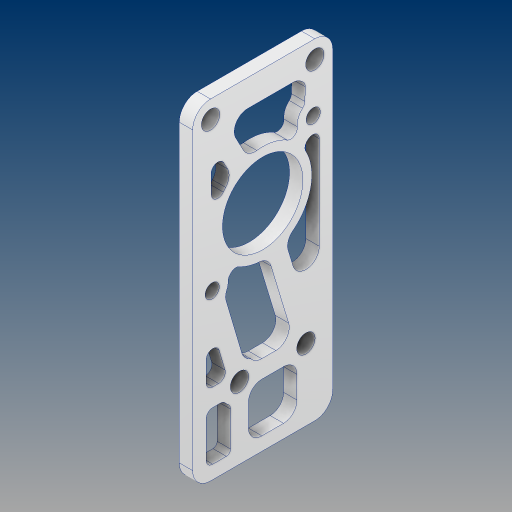
# Autodesk Inventor part: INTK_008_EncoderBracket
Saved by Autodesk Inventor 2024.3 (Build 283343000, 343)
## iProperties
Created: 2024-08-04
Part Number: INTK_008_EncoderBracket
Material: Aluminum 6061
Document SubType Name: Modeling
Designer: Kenji
Density: 2.7 g/cm^3
Appearance: Aluminum - Flat
Author: Kenji
Autodesk Inventor part; units mm, degrees
ref_plane "YZ Plane" through (0, 0, 0) normal (1, 0, 0) x (0, 1, 0)
ref_plane "XZ Plane" through (0, 0, 0) normal (0, 1, 0) x (-1, 0, 0)
ref_plane "XY Plane" through (0, 0, 0) normal (0, 0, 1) x (1, 0, 0)
sketch "Sketch1" plane through (0, 0, 0) normal (1, 0, 0) x (0, 1, 0)
  line L0 (0, 0) -> (457.2, 0) construction
  line L1 (457.2, 0) -> (457.2, 25.4) construction
  line L2 (457.2, 25.4) -> (0, 25.4) construction
  line L3 (0, 25.4) -> (0, 0) construction
  line L4 (0, 0) -> (25.4, 0) construction
  line L5 (25.4, 0) -> (25.4, -279.4) construction
  line L6 (25.4, -279.4) -> (0, -279.4) construction
  line L7 (0, -279.4) -> (0, 0) construction
  line L8 (0, 0) -> (25.4, 0) construction
  line L9 (25.4, 0) -> (25.4, -19.05) construction
  line L10 (25.4, -19.05) -> (0, -19.05) construction
  line L11 (0, -19.05) -> (0, 0) construction
  line L12 (25.4, -279.4) -> (0, -279.4) construction
  line L13 (0, -279.4) -> (0, -260.35) construction
  line L14 (0, -260.35) -> (25.4, -260.35) construction
  line L15 (25.4, -260.35) -> (25.4, -279.4) construction
  circle A0 centre (101.6254, -38.1) radius 14.2875
  line L16 (83.6649, -20.1395) -> (119.5859, -56.0605) construction
  line L17 (101.6254, -38.1) -> (101.6254, -52.3875) construction
  circle A1 centre (119.5859, -56.0605) radius 2.5019
  circle A2 centre (83.6649, -20.1395) radius 2.5019
  line L18 (25.4, -20.32) -> (57.15, -20.32) construction
  line L19 (57.15, -20.32) -> (57.15, -39.37) construction
  line L20 (57.15, -39.37) -> (25.4, -39.37) construction
  line L21 (25.4, -39.37) -> (25.4, -20.32) construction
  circle A3 centre (50.8, -29.845) radius 3.2512
  circle A4 centre (136.6774, -19.558) radius 6.35 construction
  circle A5 centre (136.6774, -19.558) radius 3.2512
  line L22 (72.9234, -13.208) -> (130.3274, -13.208) construction
  line L23 (130.3274, -13.208) -> (130.3274, -62.992) construction
  line L24 (130.3274, -62.992) -> (72.9234, -62.992) construction
  line L25 (72.9234, -62.992) -> (72.9234, -13.208) construction
  line L26 (25.4, -43.942) -> (57.15, -43.942) construction
  line L27 (57.15, -43.942) -> (57.15, -62.992) construction
  line L28 (57.15, -62.992) -> (25.4, -62.992) construction
  line L29 (25.4, -62.992) -> (25.4, -43.942) construction
  circle A6 centre (50.8, -53.467) radius 3.2512
  circle A7 centre (136.6774, -56.642) radius 6.35 construction
  circle A8 centre (136.6774, -56.642) radius 3.2512
  line L30 (136.6774, -62.992) -> (31.75, -62.992)
  line L31 (25.4, -56.642) -> (25.4, -19.558)
  line L32 (31.75, -13.208) -> (136.6774, -13.208)
  arc A9 (31.75, -13.208) -> (25.4, -19.558) centre (31.75, -19.558) ccw
  arc A10 (25.4, -56.642) -> (31.75, -62.992) centre (31.75, -56.642) ccw
  line L33 (143.0274, -19.558) -> (143.0274, -56.642)
  arc A11 (136.6774, -62.992) -> (143.0274, -56.642) centre (136.6774, -56.642) ccw
  arc A12 (143.0274, -19.558) -> (136.6774, -13.208) centre (136.6774, -19.558) ccw
  point P0 (83.6649, -17.6376)
  point P1 (101.6254, -38.1)
  point P2 (101.6254, -62.992)
  point P3 (25.4, -62.992)
  point P4 (25.4, -13.208)
  dimension "d7" = 28.575
  dimension "d14" = 5.0038
  dimension "d0" = 457.2
  dimension "d1" = 25.4
  dimension "d2" = 25.4
  dimension "d3" = 279.4
  dimension "d5" = 19.05
  dimension "d8" = 101.6254
  dimension "d9" = 38.1
  dimension "d10" = 50.8
  dimension "d11" = 25.4
  dimension "d12" = 45
  dimension "d13" = 5.0038
  dimension "d15" = 31.75
  dimension "d16" = 19.05
  dimension "d18" = 6.5024
  dimension "d19" = 9.525
  dimension "d20" = 6.35
  dimension "d27" = 12.7
  dimension "d28" = 6.5024
  dimension "d34" = 49.784
  dimension "d35" = 57.404
  dimension "d36" = 24.892
  dimension "d37" = 28.702
  dimension "d46" = 31.75
  dimension "d47" = 19.05
  dimension "d48" = 6.5024
  dimension "d49" = 9.525
  dimension "d50" = 6.35
  dimension "d51" = 12.7
  dimension "d52" = 6.5024
  dimension "d53" = 6.35
  dimension "d128" = 29.845
  dimension "d129" = 19.05
  dimension "d130" = 53.467
  constraints: 68 end point, 14 parallel, 12 point on circle, 12 point on line, 11 centre point, 10 tangent, 8 perpendicular, 7 horizontal, 6 coincident, 3 equal radius, 3 vertical alignment, 2 collinear, 2 midpoint, 2 vertical, 4 other
  measures "d0" distance of L2.end L1.end
  measures "d1" distance of L1.end L0.end
  measures "d2" distance of L5.end L6.end
  measures "d3" distance of L4.end L5.end
  measures "d5" distance of L12.end L13.end
  measures "d8" distance from line of L7 point (101.625, -38.1)
  measures "d9" distance from line of L0 point (101.625, -38.1)
  measures "d10" distance of L16.start L16.end
  measures "d11" distance of L16.end L17.start
  measures "d12" angle of L17 L16
  measures "d13" diameter of A1
  measures "d15" distance of L19.end L20.end
  measures "d16" distance of L18.end L19.end
  measures "d18" diameter of A3
  measures "d19" distance from line of L18 A3.centre
  measures "d20" distance from line of L19 A3.centre
  measures "d27" diameter of A4
  measures "d28" diameter of A5
  measures "d34" distance of L22.end L23.end
  measures "d35" distance between parallel lines of L25 L23
  measures "d36" distance of point (101.625, -62.992) point (101.625, -38.1)
  measures "d37" distance from line of L25 point (101.625, -38.1)
  measures "d46" distance of L27.end L28.end
  measures "d47" distance of L26.end L27.end
  measures "d48" diameter of A6
  measures "d49" distance from line of L26 A6.centre
  measures "d50" distance from line of L27 A6.centre
  measures "d51" diameter of A7
  measures "d52" diameter of A8
  measures "d53" radius of A9
  measures "d128" distance from line of L0 A3.centre
  measures "d129" distance between parallel lines of L0 L10
  measures "d130" distance from line of L0 A6.centre
extrude "Extrusion2" add sketch "Sketch1" along normal blind 4.7625
sketch "Sketch2" plane through (4.7625, 0, 0) normal (1, 0, 0) x (0, 0, -1)
  line L0 (13.208, 136.6774) -> (13.208, 31.75) construction
  arc A0 (13.208, 31.75) -> (19.558, 25.4) centre (19.558, 31.75) ccw construction
  line L1 (19.558, 25.4) -> (56.642, 25.4) construction
  arc A1 (56.642, 25.4) -> (62.992, 31.75) centre (56.642, 31.75) ccw construction
  line L2 (62.992, 31.75) -> (62.992, 136.6774) construction
  arc A2 (62.992, 136.6774) -> (56.642, 143.0274) centre (56.642, 136.6774) ccw construction
  line L3 (56.642, 143.0274) -> (19.558, 143.0274) construction
  arc A3 (19.558, 143.0274) -> (13.208, 136.6774) centre (19.558, 136.6774) ccw construction
  circle A4 centre (38.1, 101.6254) radius 14.2875 construction
  circle A5 centre (56.0605, 119.5859) radius 2.5019 construction
  circle A6 centre (20.1395, 83.6649) radius 2.5019 construction
  circle A7 centre (29.845, 50.8) radius 3.2512 construction
  circle A8 centre (53.467, 50.8) radius 3.2512 construction
  circle A9 centre (56.642, 136.6774) radius 3.2512 construction
  circle A10 centre (19.558, 136.6774) radius 3.2512 construction
  line L4 (19.558, 138.2522) -> (56.642, 138.2522) construction
  arc A11 (58.2168, 136.6774) -> (56.642, 138.2522) centre (56.642, 136.6774) ccw construction
  line L5 (58.2168, 136.6774) -> (58.2168, 31.75) construction
  arc A12 (56.642, 30.1752) -> (58.2168, 31.75) centre (56.642, 31.75) ccw construction
  line L6 (56.642, 30.1752) -> (19.558, 30.1752) construction
  arc A13 (17.9832, 31.75) -> (19.558, 30.1752) centre (19.558, 31.75) ccw construction
  line L7 (17.9832, 31.75) -> (17.9832, 136.6774) construction
  arc A14 (19.558, 138.2522) -> (17.9832, 136.6774) centre (19.558, 136.6774) ccw construction
  circle A15 centre (19.558, 136.6774) radius 6.4262 construction
  circle A16 centre (56.642, 136.6774) radius 6.4262 construction
  circle A17 centre (56.0605, 119.5859) radius 5.6769 construction
  circle A18 centre (38.1, 101.6254) radius 17.4625 construction
  circle A19 centre (20.1395, 83.6649) radius 5.6769 construction
  circle A20 centre (29.845, 50.8) radius 6.4262 construction
  circle A21 centre (53.467, 50.8) radius 6.4262 construction
  line L8 (22.5628, 130.997) -> (29.9347, 117.0613) construction
  line L9 (56.4235, 130.2549) -> (56.2535, 125.2595) construction
  line L10 (52.0463, 115.5717) -> (50.4479, 113.9733) construction
  line L11 (53.2364, 129.9526) -> (53.0859, 125.5295)
  line L12 (19.6285, 130.2516) -> (20.0772, 89.3414) construction
  line L13 (28.5365, 126.4943) -> (31.1955, 121.4677)
  line L14 (25.9842, 136.6774) -> (50.2158, 136.6774) construction
  line L15 (32.7576, 133.5024) -> (48.7511, 133.5024)
  arc A22 (46.8385, 116.7442) -> (35.9928, 118.9603) centre (38.1, 101.6254) ccw
  arc A23 (52.2868, 123.827) -> (50.4099, 119.0407) centre (56.0605, 119.5859) ccw
  arc A24 (24.977, 133.2233) -> (25.1451, 133.5024) centre (19.558, 136.6774) ccw
  arc A25 (52.115, 132.1164) -> (52.4191, 131.8335) centre (56.642, 136.6774) ccw
  arc A26 (52.115, 132.1164) -> (48.7511, 133.5024) centre (48.7511, 128.7272) ccw
  arc A27 (32.7576, 133.5024) -> (28.5365, 126.4943) centre (32.7576, 128.7272) ccw
  arc A28 (31.1955, 121.4677) -> (35.9928, 118.9603) centre (35.4166, 123.7006) ccw
  circle A29 centre (48.0333, 118.8113) radius 2.3876 construction
  arc A30 (46.8385, 116.7442) -> (50.4099, 119.0407) centre (48.0333, 118.8113) ccw
  circle A31 centre (50.8502, 130.0338) radius 2.3876 construction
  circle A32 centre (50.6997, 125.6107) radius 2.3876 construction
  arc A33 (53.2364, 129.9526) -> (52.4191, 131.8335) centre (50.8502, 130.0338) ccw
  arc A34 (52.2868, 123.827) -> (53.0859, 125.5295) centre (50.6997, 125.6107) ccw
  line L16 (21.7473, 78.2204) -> (28.0249, 56.9631) construction
  line L17 (47.0408, 50.8) -> (36.2712, 50.8) construction
  line L18 (51.6072, 56.9512) -> (43.1538, 84.9102) construction
  line L19 (23.4188, 50.8) -> (17.9832, 50.8) construction
  line L20 (29.845, 44.3738) -> (29.845, 30.1752) construction
  line L21 (53.467, 44.3738) -> (53.467, 30.1752) construction
  line L22 (45.5168, 47.625) -> (37.7952, 47.625)
  line L23 (33.02, 42.8498) -> (33.02, 34.9504)
  line L24 (50.292, 42.8498) -> (50.292, 34.9504)
  line L25 (20.6386, 101.4339) -> (19.9447, 101.4263) construction
  line L26 (24.2401, 121.0363) -> (25.5825, 118.4985)
  arc A35 (24.9558, 113.1219) -> (24.1124, 112.0794) centre (38.1, 101.6254) ccw
  line L27 (19.7421, 119.8937) -> (19.8124, 113.4825)
  circle A36 centre (22.1296, 119.9199) radius 2.3876 construction
  arc A37 (24.9558, 113.1219) -> (25.5825, 118.4985) centre (21.3615, 116.2657) ccw
  arc A38 (24.2401, 121.0363) -> (19.7421, 119.8937) centre (22.1296, 119.9199) ccw
  circle A39 centre (22.1999, 113.5087) radius 2.3876 construction
  arc A40 (19.8124, 113.4825) -> (24.1124, 112.0794) centre (22.1999, 113.5087) ccw
  arc A41 (33.02, 45.2129) -> (35.4321, 47.625) centre (29.845, 50.8) ccw construction
  line L28 (37.7952, 30.1752) -> (45.5168, 30.1752)
  arc A42 (33.02, 45.2129) -> (35.4321, 47.625) centre (29.845, 50.8) ccw construction
  arc A43 (47.8799, 47.625) -> (50.292, 45.2129) centre (53.467, 50.8) ccw construction
  arc A44 (37.7952, 47.625) -> (33.02, 42.8498) centre (37.7952, 42.8498) ccw
  arc A45 (50.292, 42.8498) -> (45.5168, 47.625) centre (45.5168, 42.8498) ccw
  arc A46 (33.02, 34.9504) -> (37.7952, 30.1752) centre (37.7952, 34.9504) ccw
  arc A47 (45.5168, 30.1752) -> (50.292, 34.9504) centre (45.5168, 34.9504) ccw
  line L29 (23.0204, 47.625) -> (20.3454, 47.625)
  line L30 (26.67, 43.9754) -> (26.67, 31.6738)
  line L31 (17.9832, 45.2628) -> (17.9832, 32.5374)
  line L32 (20.3454, 30.1752) -> (25.1714, 30.1752)
  circle A48 centre (25.1714, 31.6738) radius 1.4986 construction
  arc A49 (25.1714, 30.1752) -> (26.67, 31.6738) centre (25.1714, 31.6738) ccw
  arc A50 (17.9832, 32.5374) -> (20.3454, 30.1752) centre (20.3454, 32.5374) ccw
  arc A51 (24.8547, 46.7511) -> (25.7961, 45.8097) centre (29.845, 50.8) ccw
  arc A52 (24.8547, 46.7511) -> (23.0204, 47.625) centre (23.0204, 45.2628) ccw
  arc A53 (26.67, 43.9754) -> (25.7961, 45.8097) centre (24.3078, 43.9754) ccw
  arc A54 (20.3454, 47.625) -> (17.9832, 45.2628) centre (20.3454, 45.2628) ccw
  line L33 (24.1537, 87.6791) -> (25.7521, 89.2775) construction
  line L34 (26.5133, 85.5486) -> (26.8713, 85.9066)
  line L35 (47.3285, 60.1322) -> (41.0713, 80.8273)
  line L36 (25.1062, 78.0566) -> (30.6551, 59.267)
  line L37 (42.7576, 53.975) -> (37.7359, 53.975)
  arc A55 (29.7071, 86.312) -> (36.844, 84.2081) centre (38.1, 101.6254) ccw
  arc A56 (25.3245, 81.3534) -> (25.8147, 83.8025) centre (20.1395, 83.6649) ccw
  arc A57 (34.372, 55.361) -> (32.9371, 56.4334) centre (29.845, 50.8) ccw
  arc A58 (48.8109, 55.2291) -> (47.8799, 53.975) centre (53.467, 50.8) ccw construction
  arc A59 (41.0713, 80.8273) -> (36.844, 84.2081) centre (36.5005, 79.4453) ccw
  arc A60 (42.7576, 53.975) -> (47.3285, 60.1322) centre (42.7576, 58.7502) ccw
  arc A61 (34.372, 55.361) -> (37.7359, 53.975) centre (37.7359, 58.7502) ccw
  arc A62 (30.6551, 59.267) -> (32.9371, 56.4334) centre (35.2348, 60.6194) ccw
  circle A63 centre (28.5596, 84.2183) radius 2.3876 construction
  arc A64 (25.3245, 81.3534) -> (25.1062, 78.0566) centre (29.6859, 79.4091) ccw
  circle A65 centre (28.2016, 83.8603) radius 2.3876 construction
  arc A66 (29.7071, 86.312) -> (26.8713, 85.9066) centre (28.5596, 84.2183) ccw
  arc A67 (26.5133, 85.5486) -> (25.8147, 83.8025) centre (28.2016, 83.8603) ccw
  line L38 (54.1409, 113.1762) -> (53.8188, 112.8541)
  line L39 (48.8708, 76.9724) -> (47.1496, 82.665)
  line L40 (58.2168, 111.4879) -> (58.2168, 78.3544)
  arc A68 (58.2168, 55.1284) -> (54.8892, 57.0669) centre (53.467, 50.8) ccw construction
  arc A69 (48.7957, 87.8217) -> (53.4134, 110.0183) centre (38.1, 101.6254) ccw
  arc A70 (48.7957, 87.8217) -> (47.1496, 82.665) centre (51.7204, 84.047) ccw
  arc A71 (48.8708, 76.9724) -> (58.2168, 78.3544) centre (53.4416, 78.3544) ccw
  circle A72 centre (55.5071, 111.1658) radius 2.3876 construction
  circle A73 centre (55.8292, 111.4879) radius 2.3876 construction
  arc A74 (58.2168, 111.4879) -> (54.1409, 113.1762) centre (55.8292, 111.4879) ccw
  arc A75 (53.8188, 112.8541) -> (53.4134, 110.0183) centre (55.5071, 111.1658) ccw
  line L41 (22.6109, 64.086) -> (24.7016, 57.0062)
  line L42 (22.4362, 53.975) -> (20.3454, 53.975)
  line L43 (17.9832, 63.417) -> (17.9832, 56.3372)
  arc A76 (17.9832, 78.4134) -> (18.4273, 78.2523) centre (20.1395, 83.6649) ccw
  arc A77 (25.2176, 55.2591) -> (24.2579, 53.975) centre (29.845, 50.8) ccw
  arc A78 (22.4362, 53.975) -> (24.7016, 57.0062) centre (22.4362, 56.3372) ccw
  arc A79 (17.9832, 56.3372) -> (20.3454, 53.975) centre (20.3454, 56.3372) ccw
  arc A80 (22.6109, 64.086) -> (17.9832, 63.417) centre (20.3454, 63.417) ccw
  point P0 (0, 0)
  point P1 (32.8773, 118.2886)
  point P2 (51.0549, 133.5024)
  point P3 (33.02, 30.1752)
  point P4 (50.292, 30.1752)
  point P5 (27.2642, 115.3194)
  point P6 (50.292, 45.2129)
  point P7 (33.02, 30.1752)
  point P8 (24.2579, 47.625)
  point P9 (17.9832, 47.625)
  point P10 (26.67, 45.2129)
  point P11 (17.9832, 30.1752)
  point P12 (40.0305, 84.2699)
  point P13 (24.5173, 80.0508)
  point P14 (31.3076, 57.0575)
  point P15 (35.4321, 53.975)
  point P16 (46.1087, 86.1077)
  point P17 (17.9832, 53.975)
  dimension "d56" = 4.7752
  dimension "d57" = 3.175
  dimension "d58" = 3.175
  dimension "d59" = 3.175
  dimension "d60" = 3.175
  dimension "d61" = 3.175
  dimension "d62" = 3.175
  dimension "d63" = 3.175
  dimension "d65" = 3.175
  dimension "d69" = 3.175
  dimension "d70" = 3.175
  dimension "d71" = 4.7752
  dimension "d72" = 4.7752
  dimension "d73" = 4.7752
  dimension "d74" = 4.7752
  dimension "d75" = 3.175
  dimension "d76" = 3.175
  dimension "d77" = 3.175
  dimension "d79" = 3.175
  dimension "d80" = 4.7752
  dimension "d81" = 4.7752
  dimension "d82" = 4.7752
  dimension "d87" = 4.7752
  dimension "d88" = 4.7752
  dimension "d89" = 3.175
  dimension "d90" = 3.175
  dimension "d91" = 2.9972
  dimension "d92" = 2.3622
  dimension "d93" = 2.3622
  dimension "d94" = 2.3622
  dimension "d95" = 3.175
  dimension "d96" = 3.175
  dimension "d97" = 3.175
  dimension "d98" = 3.175
  dimension "d99" = 4.7752
  dimension "d100" = 4.7752
  dimension "d101" = 4.7752
  dimension "d102" = 4.7752
  dimension "d113" = 3.175
  dimension "d114" = 3.175
  dimension "d115" = 4.7752
  dimension "d116" = 4.7752
  dimension "d117" = 4.7752
  dimension "d118" = 4.7752
  dimension "d119" = 3.175
  dimension "d120" = 3.175
  dimension "d124" = 2.3622
  dimension "d125" = 2.3622
  constraints: 149 point on circle, 80 end point, 76 point on line, 71 tangent, 66 centre point, 17 parallel, 9 concentric, 9 equal radius, 5 perpendicular, 3 collinear, 2 horizontal, 1 vertical, 76 other
  measures "d56" distance between parallel lines of L3 L4
  measures "d57" radial gap between concentric circles of A10 A15
  measures "d58" radial gap between concentric circles of A9 A16
  measures "d59" radial gap between concentric circles of A5 A17
  measures "d65" distance between parallel lines of L9 L11
  measures "d69" distance between parallel lines of L8 L13
  measures "d70" distance between parallel lines of L14 L15
  measures "d71" radius of A26
  measures "d72" diameter of A29
  measures "d73" diameter of A31
  measures "d74" diameter of A32
  measures "d75" distance between parallel lines of L17 L22
  measures "d76" distance between parallel lines of L20 L23
  measures "d77" distance between parallel lines of L21 L24
  measures "d79" distance between parallel lines of L8 L26
  measures "d80" diameter of A36
  measures "d81" radius of A37
  measures "d82" diameter of A39
  measures "d87" radius of A44
  measures "d88" radius of A46
  measures "d89" distance between parallel lines of L19 L29
  measures "d90" distance between parallel lines of L20 L30
  measures "d91" diameter of A48
  measures "d92" radius of A50
  measures "d93" radius of A52
  measures "d94" radius of A54
  measures "d95" distance between parallel lines of L33 L34
  measures "d96" distance between parallel lines of L18 L35
  measures "d97" distance between parallel lines of L16 L36
  measures "d98" distance between parallel lines of L17 L37
  measures "d99" radius of A59
  measures "d100" diameter of A63
  measures "d101" radius of A64
  measures "d102" diameter of A65
  measures "d113" distance between parallel lines of L10 L38
  measures "d114" distance between parallel lines of L18 L39
  measures "d115" radius of A70
  measures "d116" radius of A71
  measures "d117" diameter of A72
  measures "d118" diameter of A73
  measures "d119" distance between parallel lines of L16 L41
  measures "d120" distance between parallel lines of L19 L42
  measures "d124" radius of A78
  measures "d125" radius of A80
extrude "Extrusion3" cut sketch "Sketch2" against normal blind 4.7625 contours L11 A34 A23 A30 A22 A28 L13 A27 L15 A26 A25 A33 | A45 L24 A47 L28 A46 L23 A44 L22 | L26 A37 A35 A40 L27 A38 | A52 A51 A53 L30 A49 L32 A50 L31 A54 L29 | L34 A66 A55 A59 L35 A60 L37 A61 A57 A62 L36 A64 A56 A67
extrude "Extrusion4" cut sketch "Sketch2" against normal blind 4.7625 contours A74 L40 A71 L39 A70 A69 A75 L38 | L41 A78 L42 A79 L43 A80
body "Solid2"
